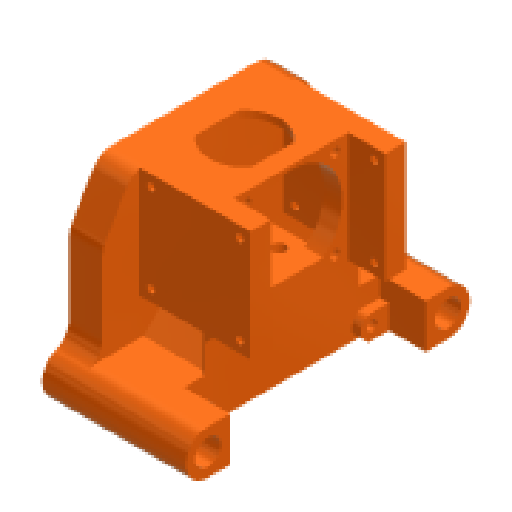
# Autodesk Inventor part: Tool_Revo
Saved by Autodesk Inventor 2023.2 (Build 272271000, 271)
## iProperties
Created: 2022-06-19
Part Number: Tool_Revo
Material: ABS Plastic
Document SubType Name: Modeling
Designer: Remo
Density: 1.06 g/cm^3
Appearance: Smooth - Light Orange
Author: Remo
Autodesk Inventor part; units mm, degrees
note: some values were not read from the file. Chosen so that the rebuilt part matches the saved one: direction of "Hole6"; direction of "Hole8".
ref_plane "YZ Plane" through (0, 0, 0) normal (1, 0, 0) x (0, 1, 0)
ref_plane "XZ Plane" through (0, 0, 0) normal (0, 1, 0) x (-1, 0, 0)
ref_plane "XY Plane" through (0, 0, 0) normal (0, 0, 1) x (1, 0, 0)
sketch "Sketch1" plane through (0, 0, 0) normal (1, 0, 0) x (0, 1, 0)
  circle A0 centre (8.9201, -5.15) radius 5.15
  circle A1 centre (8.9201, 5.15) radius 5.15
  circle A2 centre (0, 10.3) radius 5.15
  circle A3 centre (-8.9201, 5.15) radius 5.15
  circle A4 centre (-8.9201, -5.15) radius 5.15
  circle A5 centre (0, -10.3) radius 5.15
  line L0 (-27.5, 7.5) -> (-16.5, 7.5)
  line L1 (-16.5, 7.5) -> (-16.5, -7.5)
  line L2 (-16.5, -7.5) -> (-27.5, -7.5)
  line L3 (-27.5, -7.5) -> (-27.5, 7.5)
  line L4 (-27.5, 7.5) -> (-16.5, -7.5) construction
  line L5 (-16.5, 7.5) -> (-27.5, -7.5) construction
  line L6 (14.7452, -10.5394) -> (20.2452, -20.0657)
  line L7 (1.7548, -18.0394) -> (14.7452, -10.5394)
  line L8 (7.2548, -27.5657) -> (1.7548, -18.0394)
  line L9 (20.2452, -20.0657) -> (7.2548, -27.5657)
  line L10 (1.7548, 18.0394) -> (7.2548, 27.5657)
  line L11 (14.7452, 10.5394) -> (1.7548, 18.0394)
  line L12 (20.2452, 20.0657) -> (14.7452, 10.5394)
  line L13 (7.2548, 27.5657) -> (20.2452, 20.0657)
  arc A6 (-22, 31) -> (-28, 25) centre (-22, 25) ccw
  arc A7 (-28, -25) -> (-22, -31) centre (-22, -25) ccw
  line L14 (-28, 25) -> (-28, -25)
  line L15 (-22, 31) -> (10, 31)
  line L16 (10, -31) -> (-22, -31)
  line L17 (10, -31) -> (24, -22.9171)
  line L18 (24, -22.9171) -> (24, 22.9171)
  line L19 (24, 22.9171) -> (10, 31)
  circle A8 centre (-22, -32.5) radius 3.5
  circle A9 centre (-22, 32.5) radius 3.5
  arc A10 (-26.6837, -28.75) -> (-16.1905, -31) centre (-22, -32.5) ccw
  arc A11 (-16.1905, 31) -> (-26.6837, 28.75) centre (-22, 32.5) ccw
  line L20 (-28, -32.5) -> (-28, -25)
  line L21 (-28, 32.5) -> (-28, 25)
  point P0 (0, 0)
  point P1 (-22, 0)
  point P2 (-4.46, -7.725)
  point P3 (-8.9201, 0)
  point P4 (-4.46, 7.725)
  point P5 (4.46, 7.725)
  point P6 (8.9201, 0)
  point P7 (4.46, -7.725)
  dimension "d0" = 10.3
  dimension "d3" = 360
  dimension "d5" = 15
  dimension "d6" = 11
  dimension "d7" = 22
  dimension "d10" = 360
  dimension "d15" = 12
  dimension "d29" = 10
  dimension "d31" = 24
  dimension "d135" = 50
  dimension "d136" = 52
  dimension "d137" = 25
  dimension "d138" = 65
  dimension "d139" = 32.5
  dimension "d140" = 7
  constraints: 44 end point, 13 point on circle, 12 centre point, 9 tangent, 4 equal radius, 4 parallel, 3 horizontal, 3 point on line, 3 vertical, 2 coincident, 2 midpoint, 2 vertical alignment, 1 collinear, 1 horizontal alignment, 1 perpendicular, 38 other
  measures "d0" diameter of A0
  measures "d5" distance of L2.end L0.start
  measures "d6" distance of L1.end L2.end
  measures "d7" distance of point (-22, 0) point (0, 0)
  measures "d15" diameter of A6
  measures "d29" horizontal distance of L16.start point (0, 0)
  measures "d31" distance from line of point (0, 0) L18
  measures "d135" distance of A6.centre A7.centre
  measures "d136" distance between parallel lines of L18 L14
  measures "d137" vertical distance of A6.centre point (0, 0)
  measures "d138" distance of A9.centre A8.centre
  measures "d139" distance of point (-22, 0) A9.centre
  measures "d140" diameter of A8
extrude "Layer1_Magnets_16" add sketch "Sketch1" along normal blind 1.6 contours A0 A5 A4 A3 A2 A1 | A6 A9 L15 L19 L18 L17 L16 A8 A7 L14 | A11 L15 A9 A6 | A6 L21 A11 | A7 A10 L20 | A7 A8 L16 A10
sketch "Sketch2" plane through (1.6, 0, 0) normal (1, 0, 0) x (0, 0, -1)
  line L0 (-32.5, -28) -> (32.5, -28) projected
  line L1 (31, -16.1905) -> (31, 10) projected
  line L2 (-31, 10) -> (-31, -16.1905) projected
  arc A0 (7.725, -4.46) -> (7.725, 4.46) centre (10.3, 0) ccw projected
  arc A1 (0, -8.9201) -> (7.725, -4.46) centre (5.15, -8.9201) ccw projected
  arc A2 (-7.725, -4.46) -> (0, -8.9201) centre (-5.15, -8.9201) ccw projected
  arc A3 (-7.725, 4.46) -> (-7.725, -4.46) centre (-10.3, 0) ccw projected
  arc A4 (0, 8.9201) -> (-7.725, 4.46) centre (-5.15, 8.9201) ccw projected
  arc A5 (7.725, 4.46) -> (0, 8.9201) centre (5.15, 8.9201) ccw projected
  line L3 (-18.0394, 1.7548) -> (-27.5657, 7.2548) projected
  line L4 (-27.5657, 7.2548) -> (-20.0657, 20.2452) projected
  line L5 (-20.0657, 20.2452) -> (-10.5394, 14.7452) projected
  line L6 (-10.5394, 14.7452) -> (-18.0394, 1.7548) projected
  line L7 (10.5394, 14.7452) -> (20.0657, 20.2452) projected
  line L8 (20.0657, 20.2452) -> (27.5657, 7.2548) projected
  line L9 (27.5657, 7.2548) -> (18.0394, 1.7548) projected
  line L10 (18.0394, 1.7548) -> (10.5394, 14.7452) projected
  line L11 (-7.5, -27.5) -> (-7.5, -16.5) projected
  line L12 (-7.5, -16.5) -> (7.5, -16.5) projected
  line L13 (7.5, -16.5) -> (7.5, -27.5) projected
  line L14 (7.5, -27.5) -> (-7.5, -27.5) projected
  arc A6 (0, 8.9201) -> (7.725, 4.46) centre (5.15, 8.9201) ccw projected
  arc A7 (-7.725, 4.46) -> (0, 8.9201) centre (-5.15, 8.9201) ccw projected
  arc A8 (-7.725, -4.46) -> (-7.725, 4.46) centre (-10.3, 0) ccw projected
  arc A9 (0, -8.9201) -> (-7.725, -4.46) centre (-5.15, -8.9201) ccw projected
  arc A10 (7.725, -4.46) -> (0, -8.9201) centre (5.15, -8.9201) ccw projected
  arc A11 (7.725, 4.46) -> (7.725, -4.46) centre (10.3, 0) ccw projected
  line L15 (31, 10) -> (22.9171, 24) projected
  line L16 (22.9171, 24) -> (-22.9171, 24) projected
  line L17 (-22.9171, 24) -> (-31, 10) projected
  arc A12 (32.5, -28) -> (31, -16.1905) centre (32.5, -22) ccw projected
  arc A13 (-31, -16.1905) -> (-32.5, -28) centre (-32.5, -22) ccw projected
  circle A14 centre (-32.5, -22) radius 3.5 projected
  circle A15 centre (32.5, -22) radius 3.5 projected
  point P0 (0, 0)
  point P1 (-7.725, 4.46)
  point P2 (-7.725, 4.46)
  point P3 (-7.725, 4.46)
  point P4 (-7.725, 4.46)
  point P5 (-7.725, -4.46)
  point P6 (-7.725, -4.46)
  point P7 (-7.725, -4.46)
  point P8 (-7.725, -4.46)
  point P9 (0, -8.9201)
  point P10 (0, -8.9201)
  point P11 (0, -8.9201)
  point P12 (0, -8.9201)
  point P13 (7.725, -4.46)
  point P14 (7.725, -4.46)
  point P15 (7.725, -4.46)
  point P16 (7.725, -4.46)
  point P17 (7.725, 4.46)
  point P18 (7.725, 4.46)
  point P19 (7.725, 4.46)
  point P20 (7.725, 4.46)
  point P21 (0, 8.9201)
  point P22 (0, 8.9201)
  point P23 (0, 8.9201)
  point P24 (0, 8.9201)
extrude "Layer2_Coupler_80" add sketch "Sketch2" along normal blind 6.4 contours A13 L2 L17 L16 L15 L1 A12 L0 | A11 A0 | A1 A10 | A10 A9 A8 A7 A6 A11 | A6 A5 | A2 A9 | A7 A4 | A3 A8
sketch "Sketch3" plane through (8, 0, 0) normal (1, 0, 0) x (0, 0, -1)
  line L0 (-18.0394, 1.7548) -> (-27.5657, 7.2548) projected
  line L1 (-27.5657, 7.2548) -> (-20.0657, 20.2452) projected
  line L2 (-20.0657, 20.2452) -> (-10.5394, 14.7452) projected
  line L3 (-10.5394, 14.7452) -> (-18.0394, 1.7548) projected
  line L4 (10.5394, 14.7452) -> (20.0657, 20.2452) projected
  line L5 (20.0657, 20.2452) -> (27.5657, 7.2548) projected
  line L6 (27.5657, 7.2548) -> (18.0394, 1.7548) projected
  line L7 (18.0394, 1.7548) -> (10.5394, 14.7452) projected
  line L8 (-7.5, -27.5) -> (-7.5, -16.5) projected
  line L9 (-7.5, -16.5) -> (7.5, -16.5) projected
  line L10 (7.5, -16.5) -> (7.5, -27.5) projected
  line L11 (7.5, -27.5) -> (-7.5, -27.5) projected
  line L12 (-32.5, -28) -> (32.5, -28) projected
  line L13 (31, -16.1905) -> (31, 10) projected
  line L14 (-31, 10) -> (-31, -16.1905) projected
  line L15 (22.9171, 24) -> (-22.9171, 24) projected
  line L16 (-22.9171, 24) -> (-31, 10) projected
  line L17 (31, 10) -> (22.9171, 24) projected
  arc A0 (-31, -16.1905) -> (-32.5, -28) centre (-32.5, -22) ccw projected
  arc A1 (32.5, -28) -> (31, -16.1905) centre (32.5, -22) ccw projected
  circle A2 centre (-32.5, -22) radius 3.5 projected
  circle A3 centre (32.5, -22) radius 3.5 projected
  point P0 (0, 0)
extrude "Layer3_Cover_90" add sketch "Sketch3" along normal blind 1 contours L0 L1 L2 L3 | L4 L5 L6 L7 | L8 L9 L10 L11 | A0 L14 L16 L15 L17 L13 A1 L12
chamfer "CouplerL" distance 7.5 angle 45 6 edges at (8, -22, 7.5) (8, -22, -7.5) (8, 4.5048, -22.8026) (8, 17.4952, -15.3026) (8, 17.4952, 15.3026) (8, 4.5048, 22.8026)
fillet "EdgeRadius" radius 6 6 edges at (4.5, 10, -31) (4.5, 10, 31) (4.5, 24, 22.9171) (4.5, 24, -22.9171) (4.5, -16.1905, 31) (4.5, -16.1905, -31)
sketch "Sketch23" plane through (9, 0, 0) normal (1, 0, 0) x (0, 0, -1)
  line L0 (19.453, 24) -> (-19.453, 24) projected
  arc A0 (-19.453, 24) -> (-24.6491, 21) centre (-19.453, 18) ccw projected
  line L1 (-24.6491, 21) -> (-30.1962, 11.3923) projected
  arc A1 (-30.1962, 11.3923) -> (-31, 8.3923) centre (-25, 8.3923) ccw projected
  line L2 (-31, 8.3923) -> (-31, -10.8757) projected
  line L3 (-32.5, -28) -> (32.5, -28) projected
  line L4 (31, -10.8757) -> (31, 8.3923) projected
  arc A2 (31, 8.3923) -> (30.1962, 11.3923) centre (25, 8.3923) ccw projected
  line L5 (30.1962, 11.3923) -> (24.6491, 21) projected
  arc A3 (24.6491, 21) -> (19.453, 24) centre (19.453, 18) ccw projected
  line L6 (33.8789, -16) -> (-33.8789, -16)
  arc A4 (-34.75, -16.4379) -> (-32.5, -28) centre (-32.5, -22) ccw projected
  arc A5 (32.5, -28) -> (34.75, -16.4379) centre (32.5, -22) ccw projected
  arc A6 (-34.75, -16.4379) -> (-31, -10.8757) centre (-37, -10.8757) ccw projected
  arc A7 (31, -10.8757) -> (34.75, -16.4379) centre (37, -10.8757) ccw projected
  circle A8 centre (32.5, -22) radius 3.5 projected
  circle A9 centre (-32.5, -22) radius 3.5 projected
  circle A10 centre (32.5, -22) radius 6
  arc A11 (32.5, -28) -> (34.75, -16.4379) centre (32.5, -22) ccw projected
  circle A12 centre (-32.5, -22) radius 6
  line L7 (20, -16) -> (10, -6)
  line L8 (10, -6) -> (-10, -6)
  line L9 (-10, -6) -> (-20, -16)
  line L10 (10, -6) -> (10, -2)
  line L11 (10, -2) -> (-10, -2)
  line L12 (-10, -2) -> (-10, -6)
  point P0 (0, 0)
  point P1 (32.5, -16)
  point P2 (-32.5, -16)
  point P3 (0, -6)
  dimension "d142" = 20
  dimension "d143" = 10
  dimension "d190" = 4
  constraints: 14 end point, 4 perpendicular, 2 centre point, 2 coincident, 2 concentric, 2 point on circle, 2 point on line, 1 horizontal, 1 midpoint, 1 tangent, 1 vertical, 1 vertical alignment
  measures "d142" distance of L7.end L8.end
  measures "d143" distance between parallel lines of L6 L8
  measures "d190" distance of L7.end L10.end
extrude "Top_Hotend" add sketch "Sketch23" along normal blind 30 contours A10 L3 A12 L6 | A10 A5 | A12 A4 | L6 L9 L8 L7 | L8 L12 L11 L10
sketch "Sketch28" plane through (39, 0, 0) normal (1, 0, 0) x (0, 0, -1)
  line L0 (-10, -6) -> (-20, -16) projected
  line L1 (-20, -16) -> (-32.5, -16) projected
  arc A0 (-32.5, -16) -> (-32.5, -28) centre (-32.5, -22) ccw projected
  line L2 (-32.5, -28) -> (32.5, -28) projected
  arc A1 (32.5, -28) -> (32.5, -16) centre (32.5, -22) ccw projected
  line L3 (32.5, -16) -> (20, -16) projected
  line L4 (20, -16) -> (10, -6) projected
  circle A2 centre (-32.5, -22) radius 3.5 projected
  circle A3 centre (32.5, -22) radius 3.5 projected
  line L5 (-32.5, -28) -> (32.5, -28) projected
  line L6 (26.5, -28) -> (26.5, -16)
  line L7 (-20, -16) -> (-32.5, -16) projected
  line L8 (-26.5, -16) -> (-26.5, -28)
  line L9 (10, -6) -> (10, -2) projected
  line L10 (10, -2) -> (-10, -2) projected
  line L11 (-10, -2) -> (-10, -6) projected
  point P0 (0, 0)
  point P1 (-26.5, -22)
  dimension "d150" = 6
  dimension "d151" = 6
  constraints: 4 end point, 4 point on line, 2 perpendicular, 1 midpoint
  measures "d150" distance from line of A1.centre L6
  measures "d151" distance of A0.centre point (-26.5, -22)
extrude "Top_EBB36" cut sketch "Sketch28" against normal blind 13 contours L11 L10 L9 L4 L3 L6 L2 L8 L1 L0 | A3
sketch "Sketch29" plane through (26, 0, 0) normal (1, 0, 0) x (0, 0, -1)
  line L0 (-26.5, -16) -> (-20, -16) projected
  line L1 (-26.5, -28) -> (-26.5, -16) projected
  line L2 (26.5, -28) -> (-26.5, -28) projected
  line L3 (20, -16) -> (26.5, -16) projected
  line L4 (10, -6) -> (20, -16) projected
  line L5 (-20, -16) -> (-10, -6) projected
  circle A0 centre (21.92, -24.5) radius 1.75 projected
  circle A1 centre (-21.92, -24.5) radius 1.75 projected
  circle A2 centre (-21.92, -24.5) radius 1.4
  circle A3 centre (-21.92, -24.5) radius 3
  circle A4 centre (21.92, -24.5) radius 1.4
  circle A5 centre (21.92, -24.5) radius 3
  line L6 (21.92, -21.5) -> (26.5, -21.5)
  line L7 (26.5, -16) -> (26.5, -28) projected
  line L8 (18.92, -24.5) -> (18.92, -28)
  line L9 (26.5, -28) -> (-26.5, -28) projected
  line L10 (-18.92, -24.5) -> (-18.92, -28)
  line L11 (-21.92, -21.5) -> (-26.5, -21.5)
  line L12 (10, -2) -> (10, -6) projected
  line L13 (-10, -2) -> (10, -2) projected
  line L14 (-10, -6) -> (-10, -2) projected
  line L15 (26.5, -16) -> (26.5, -28) projected
  point P0 (0, 0)
  point P1 (32.5, -28)
  dimension "d154" = 2.8
  dimension "d155" = 6
  constraints: 8 end point, 6 point on line, 4 centre point, 4 coincident, 4 point on circle, 2 equal radius, 2 perpendicular, 1 tangent
  measures "d154" diameter of A4
  measures "d155" diameter of A5
extrude "Top_EBB36_Mount" add sketch "Sketch29" along normal blind 3 contours L11 A3 L10 L2 L1 | A3 | L8 A5 L6 L7 L2 | A5 | A0 | A1
sketch "Sketch30" plane through (0, -28, -32.5) normal (0, -1, 0) x (1, 0, 0)
  line L0 (9, 13.047) -> (9, 51.953) projected
  line L1 (9, 57.1491) -> (9, 51.953) projected
  line L2 (9, 57.1491) -> (9, 62.6962) projected
  line L3 (9, 63.5) -> (9, 62.6962) projected
  line L4 (9, 67.25) -> (9, 63.5) projected
  line L5 (9, 67.25) -> (9, 65) projected
  line L6 (9, 65) -> (9, 52.5) projected
  line L7 (9, 52.5) -> (9, 42.5) projected
  line L8 (9, 22.5) -> (9, 12.5) projected
  line L9 (9, 12.5) -> (9, 0) projected
  line L10 (9, 0) -> (9, -2.25) projected
  line L11 (9, 1.5) -> (9, -2.25) projected
  line L12 (9, 2.3038) -> (9, 1.5) projected
  line L13 (9, 2.3038) -> (9, 7.8509) projected
  line L14 (9, 13.047) -> (9, 7.8509) projected
  line L15 (9, 42.5) -> (9, 22.5) projected
  point P0 (0, 32.5)
  point P1 (12.25, 27.5)
  point P2 (20.75, 27.5)
  point P3 (20.75, 37.5)
  point P4 (12.25, 37.5)
  dimension "d158" = 10
  dimension "d159" = 5
  dimension "d160" = 8.5
  constraints: 2 horizontal alignment, 2 vertical alignment
  measures "d158" distance of point (12.25, 37.5) point (12.25, 27.5)
  measures "d159" vertical distance of point (12.25, 27.5) point (0, 32.5)
  measures "d160" distance of point (12.25, 27.5) point (20.75, 27.5)
hole "Hotend Bolt Holes" at (12.25, -28, -5) at (20.75, -28, -5) at (20.75, -28, 5) at (12.25, -28, 5) direction (0, 1, 0) diameter 3.6 end through all counterbore diameter 6.5 counterbore depth 17 clearance for "Socket Head Cap Screw ISO 4762" size "M3" standard "ISO"
sketch "Sketch31" plane through (0, -28, -32.5) normal (0, -1, 0) x (1, 0, 0)
  circle A0 centre (20.75, 37.5) radius 3.25 projected
  circle A1 centre (12.25, 27.5) radius 3.25 projected
  circle A2 centre (20.75, 27.5) radius 3.25 projected
  circle A3 centre (12.25, 37.5) radius 3.25 projected
  line L0 (29, 59) -> (29, 51.42) projected
  line L1 (29, 59) -> (39, 59) projected
  line L2 (39, 65) -> (39, 59) projected
  line L3 (0, 65) -> (39, 65) projected
  line L4 (0, 65) -> (0, 0) projected
  line L5 (0, 0) -> (39, 0) projected
  line L6 (39, 6) -> (29, 6) projected
  line L7 (39, 6) -> (39, 0) projected
  line L8 (29, 13.58) -> (29, 6) projected
  line L9 (26, 13.58) -> (29, 13.58) projected
  line L10 (26, 13.58) -> (26, 51.42) projected
  line L11 (26, 51.42) -> (29, 51.42) projected
  point P0 (0, 32.5)
  point P1 (16.5, 32.5)
  point P2 (0, 32.5)
  dimension "d169" = 8.5
  dimension "d170" = 4.25
  constraints: 1 horizontal alignment, 1 midpoint
  measures "d169" distance of A1.centre A2.centre
  measures "d170" horizontal distance of A1.centre point (16.5, 32.5)
hole "Hotend Bowden Hole" at (16.5, -28, 0) direction (0, 1, 0) diameter 4.2 end through all
sketch "Sketch32" plane through (0, 24, 19.453) normal (0, 1, 0) x (1, 0, 0)
  line L0 (9.5, 23.3286) -> (9.5, 15.5774)
  line L1 (12.0396, 11.1787) -> (9.5, 15.5774)
  arc A0 (12.0396, 11.1787) -> (20.9604, 11.1787) centre (16.5, 19.453) ccw
  line L2 (23.5, 15.5774) -> (20.9604, 11.1787)
  line L3 (23.5, 15.5774) -> (23.5, 23.3286)
  line L4 (20.9604, 27.7273) -> (23.5, 23.3286)
  arc A1 (20.9604, 27.7273) -> (12.0396, 27.7273) centre (16.5, 19.453) ccw
  line L5 (9.5, 23.3286) -> (12.0396, 27.7273)
  circle A2 centre (16.5, 19.453) radius 3.87
  line L6 (29, 31.453) -> (29, 7.453)
  line L7 (29, 7.453) -> (29, 4.453)
  line L8 (29, 34.453) -> (29, 31.453)
  line L9 (39, -1.547) -> (9, -1.547)
  line L10 (9, -13.047) -> (9, -0.547)
  line L11 (9, 38.906) -> (9, 0)
  line L12 (9, 0) -> (9, -5.1962)
  line L13 (9, 44.1021) -> (9, 38.906)
  line L14 (9, 40.453) -> (9, 50.453)
  line L15 (37.6, -1.547) -> (10.4, -1.547)
  line L16 (10.4, 40.453) -> (37.6, 40.453)
  line L17 (9, 40.453) -> (39, 40.453)
  line L18 (39, -1.547) -> (39, 1.453)
  line L19 (39, 1.453) -> (9, 1.453)
  line L20 (39, 40.453) -> (39, 37.453)
  line L21 (39, 37.453) -> (9, 37.453)
  line L22 (29, 34.453) -> (29, 37.453)
  line L23 (29, 4.453) -> (29, 1.453)
  line L24 (24, 37.453) -> (24, 1.453)
  point P0 (0, 19.453)
extrude "Fans Sidewalls" add sketch "Sketch32" against normal blind 30 contours L6 L7 L23 L19 L24 L21 L22 L8 | L21 L11 L13 L17 L16 L20 | L19 L18 L9 L10 L12 L11
sketch "Sketch33" plane through (26, 0, 0) normal (1, 0, 0) x (0, 0, -1)
  line L0 (-26.5, -21.5) -> (-21.92, -21.5) projected
  arc A0 (-18.92, -24.5) -> (-21.92, -21.5) centre (-21.92, -24.5) ccw projected
  line L1 (-18.92, -24.5) -> (-18.92, -28) projected
  line L2 (18.92, -28) -> (-18.92, -28) projected
  line L3 (18.92, -28) -> (18.92, -24.5) projected
  arc A1 (21.92, -21.5) -> (18.92, -24.5) centre (21.92, -24.5) ccw projected
  line L4 (21.92, -21.5) -> (26.5, -21.5) projected
  line L5 (20, -16) -> (26.5, -16) projected
  line L6 (10, -6) -> (20, -16) projected
  line L7 (-20, -16) -> (-10, -6) projected
  line L8 (-26.5, -16) -> (-20, -16) projected
  line L9 (-26.5, -21.5) -> (-26.5, -16) projected
  line L10 (-18, -6) -> (-21, -6) projected
  line L11 (-26.5, -16) -> (-32.5, -16) projected
  line L12 (21, 23.7971) -> (21, -6) projected
  line L13 (20, -16) -> (32.5, -16) projected
  line L14 (-21, -6) -> (-21, -16)
  line L15 (21, -6) -> (18, -6) projected
  line L16 (21, -6) -> (21, -16)
  line L17 (20, -16) -> (26.5, -16) projected
  line L18 (18, -6) -> (-18, -6) projected
  line L19 (10, -6) -> (-10, -6) projected
  line L20 (26.5, -21.5) -> (26.5, -16) projected
  point P0 (0, 0)
  constraints: 4 end point, 2 point on line, 1 perpendicular, 1 vertical
extrude "Extrusion26" add sketch "Sketch33" along normal blind 0.6
sketch "Sketch35" plane through (29, 24, 18) normal (1, 0, 0) x (0, 0, -1)
  line L0 (0, 0) -> (36, 0) projected
  line L1 (0, 0) -> (0, -30) projected
  line L2 (36, -30) -> (0, -30) projected
  line L3 (36, 0) -> (36, -30) projected
  circle A0 centre (18, -15) radius 14
  line L4 (36, 0) -> (36, -30) projected
  line L5 (36, -30) -> (0, -30) projected
  circle A1 centre (30, -3) radius 1.25
  circle A2 centre (30, -27) radius 1.25
  circle A3 centre (6, -3) radius 1.25
  circle A4 centre (6, -27) radius 1.25
  line L6 (8, -26) -> (28, -26) projected
  point P0 (18, -24)
  point P1 (36, -15)
  point P2 (18, -30)
  point P3 (9.3397, -26)
  point P4 (26.6603, -26)
  dimension "d191" = 28
  dimension "d194" = 24
  dimension "d197" = 24
  dimension "d200" = 12
  dimension "d201" = 12
  dimension "d202" = 2.5
  constraints: 5 centre point, 2 midpoint, 1 horizontal, 1 horizontal alignment, 1 vertical, 1 vertical alignment, 6 other
  measures "d191" diameter of A0
  measures "d194" distance of A1.centre A2.centre
  measures "d197" distance of A1.centre A3.centre
  measures "d200" horizontal distance of A0.centre A1.centre
  measures "d201" horizontal distance of A1.centre A0.centre
  measures "d202" diameter of A1
extrude "HE_FAN Cut" cut sketch "Sketch35" against normal up to surface (5 mm away) contours A0 L6 | A1 | A2 | A3 | A4 picked at (19.4131, -16.9743)
chamfer "Chamfer4" distance 2.4 angle 45 1 edges at (26.6, -6, 0)
sketch "Sketch36" plane through (29, 24, 18) normal (1, 0, 0) x (0, 0, -1)
  circle A0 centre (6, -27) radius 1.25 projected
  arc A1 (26.6603, -26) -> (9.3397, -26) centre (18, -15) ccw projected
  line L0 (26.6603, -26) -> (9.3397, -26) projected
  circle A2 centre (30, -3) radius 1.25 projected
  circle A3 centre (30, -27) radius 1.25 projected
  circle A4 centre (6, -3) radius 1.25 projected
  line L1 (0, 0) -> (36, 0) projected
  line L2 (0, 0) -> (0, -30) projected
  line L3 (36, -30) -> (0, -30) projected
  line L4 (36, 0) -> (36, -30) projected
  line L5 (33.5, -30) -> (33.5, 0)
  line L6 (0, 0) -> (36, 0) projected
  line L7 (2.5, -30) -> (2.5, 0)
  point P0 (18, -24)
  point P1 (2.5, 0)
  dimension "d208" = 15.5
  dimension "d209" = 15.5
  constraints: 4 end point, 4 point on line, 2 perpendicular
  measures "d208" distance from line of L7 A1.centre
  measures "d209" distance from line of L5 A1.centre
extrude "Extrusion29" add sketch "Sketch36" along normal up to surface (10 mm away) contours L1 L7 L3 L2 | L1 L4 L3 L5
sketch "Sketch37" plane through (0, -28, -32.5) normal (0, -1, 0) x (1, 0, 0)
  circle A0 centre (16.5, 32.5) radius 2.1 projected
  circle A1 centre (20.75, 37.5) radius 3.25 projected
  circle A2 centre (12.25, 27.5) radius 3.25 projected
  circle A3 centre (20.75, 27.5) radius 3.25 projected
  circle A4 centre (12.25, 37.5) radius 3.25 projected
  line L0 (39, 6) -> (29, 6) projected
  line L1 (29, 13.58) -> (29, 6) projected
  line L2 (26.6, 13.58) -> (29, 13.58) projected
  line L3 (26.6, 51.42) -> (26.6, 13.58) projected
  line L4 (26.6, 51.42) -> (29, 51.42) projected
  line L5 (29, 59) -> (29, 51.42) projected
  line L6 (29, 59) -> (39, 59) projected
  line L7 (39, 65) -> (39, 59) projected
  line L8 (0, 65) -> (39, 65) projected
  line L9 (0, 65) -> (0, 0) projected
  line L10 (0, 0) -> (39, 0) projected
  line L11 (39, 6) -> (39, 0) projected
  circle A5 centre (16.5, 32.5) radius 4.75
  point P0 (0, 32.5)
  dimension "d215" = 9.5
  constraints: 1 centre point, 1 coincident
  measures "d215" diameter of A5
extrude "Extrusion30" cut sketch "Sketch37" against normal blind 10 contours A5 A1 | A1 A5 A3 A2 A4 | A4 A5 | A5 A3 | A2 A5 picked at (19.62, 35.3998) picked at (14.1407, 36.0464) picked at (19.62, 29.6002) picked at (14.1407, 28.9536)
sketch "Sketch39" plane through (0, 24, 19.453) normal (0, 1, 0) x (1, 0, 0)
  line L0 (0, 38.906) -> (9, 38.906) projected
  line L1 (0, 38.906) -> (0, 0) projected
  line L2 (9, 0) -> (0, 0) projected
  line L3 (9, 0) -> (9, -1.547) projected
  line L4 (9, -1.547) -> (39, -1.547) projected
  line L5 (39, -1.547) -> (39, 3.953) projected
  line L6 (29, 3.953) -> (39, 3.953) projected
  line L7 (29, 3.953) -> (29, 34.953) projected
  line L8 (29, 34.953) -> (39, 34.953) projected
  line L9 (39, 34.953) -> (39, 40.453) projected
  line L10 (39, 40.453) -> (9, 40.453) projected
  line L11 (9, 40.453) -> (9, 38.906) projected
  line L12 (9, 37.453) -> (24, 37.453) projected
  line L13 (24, 37.453) -> (24, 1.453) projected
  line L14 (24, 1.453) -> (9, 1.453) projected
  line L15 (9, 37.453) -> (9, 1.453) projected
  arc A0 (12.0396, 11.1787) -> (20.9604, 11.1787) centre (16.5, 19.453) ccw projected
  arc A1 (20.9604, 27.7273) -> (12.0396, 27.7273) centre (16.5, 19.453) ccw projected
  circle A2 centre (16.5, 19.453) radius 9.5
  point P0 (0, 19.453)
  point P1 (24, 13.622)
  point P2 (9, 13.622)
  point P3 (9, 25.2839)
  point P4 (24, 25.2839)
  dimension "d222" = 19
  constraints: 1 centre point, 1 coincident
  measures "d222" diameter of A2
extrude "Extrusion31" add sketch "Sketch39" against normal blind 2 contours L12 L13 A2 L15 | A2 L13 L14 L15
chamfer "Chamfer6" distance 2 angle 45 2 edges at (27.8, -28, 18.92) (27.8, -28, -18.92)
sketch "Sketch40" plane through (39, 24, -21) normal (0, 0, -1) x (-1, 0, 0)
  circle A0 centre (27, -3) radius 1.7 projected
  circle A1 centre (3, -27) radius 1.7 projected
  circle A2 centre (3, -3) radius 1.7 projected
  circle A3 centre (27, -27) radius 1.7 projected
  point P0 (39, -24)
hole "Hole6" at (12, 21, -21) at (36, -3, -21) at (36, 21, -21) at (12, -3, -21) direction (0, 0, 1) diameter 2 depth 5.5
sketch "Sketch42" plane through (9, 24, 21) normal (0, 0, 1) x (1, 0, 0)
  circle A0 centre (27, -3) radius 1 projected
  circle A1 centre (3, -3) radius 1 projected
  circle A2 centre (27, -27) radius 1 projected
  circle A3 centre (3, -27) radius 1 projected
  line L0 (30, 0) -> (0, 0) projected
  line L1 (30, 0) -> (30, -30) projected
  line L2 (20, -30) -> (30, -30) projected
  line L3 (17.6, -32.4) -> (20, -30) projected
  line L4 (17.6, -40) -> (17.6, -32.4) projected
  line L5 (17, -40) -> (17.6, -40) projected
  line L6 (17, -40) -> (17, -30) projected
  line L7 (0, -30) -> (17, -30) projected
  line L8 (0, -0.2029) -> (0, -30) projected
  line L9 (0, 0) -> (0, -0.2029) projected
  point P0 (-9, -24)
hole "Hole8" at (12, -3, 21) at (12, 21, 21) at (36, 21, 21) at (36, -3, 21) direction (0, 0, -1) diameter 2 depth 5.5
sketch "Sketch41" plane through (29, 0, 0) normal (1, 0, 0) x (0, 0, -1)
  circle A0 centre (-21.92, -24.5) radius 1.4 projected
  line L0 (-18.92, -26) -> (-20.92, -28) projected
  line L1 (-18.92, -26) -> (-18.92, -24.5) projected
  arc A1 (-18.92, -24.5) -> (-21.92, -21.5) centre (-21.92, -24.5) ccw projected
  line L2 (-21.92, -21.5) -> (-26.5, -21.5) projected
  line L3 (-26.5, -28) -> (-26.5, -21.5) projected
  line L4 (-26.5, -28) -> (-20.92, -28) projected
  line L5 (20.92, -28) -> (18.92, -26) projected
  line L6 (20.92, -28) -> (26.5, -28) projected
  line L7 (26.5, -21.5) -> (26.5, -28) projected
  line L8 (26.5, -21.5) -> (21.92, -21.5) projected
  arc A2 (21.92, -21.5) -> (18.92, -24.5) centre (21.92, -24.5) ccw projected
  line L9 (18.92, -24.5) -> (18.92, -26) projected
  circle A3 centre (21.92, -24.5) radius 1.4 projected
  point P0 (0, 0)
equation "\"d137\" = 0.5 * d135"
equation "\"d139\" = 0.5 * d138"
body "Solid1"
